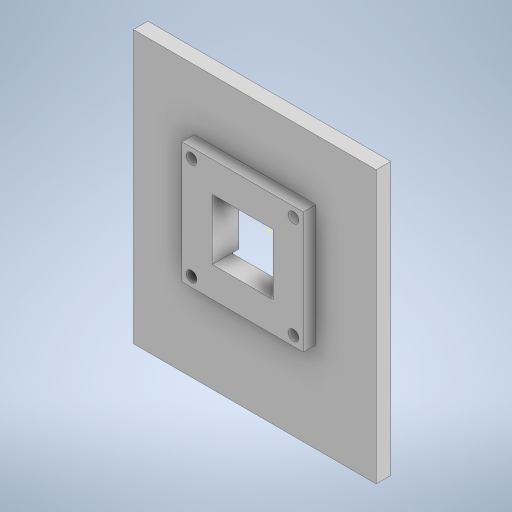
# Autodesk Inventor part: 11
Saved by Autodesk Inventor 2024 (Build 280153000, 153)
## iProperties
Created: 2025-12-09
Part Number: 11
Material: 常规
Document SubType Name: Modeling
Designer: 29555
Density: 1 g/cm^3
Appearance: 默认
Author: 29555
Autodesk Inventor part; units mm, degrees
ref_plane "YZ Plane" through (0, 0, 0) normal (1, 0, 0) x (0, 1, 0)
ref_plane "XZ Plane" through (0, 0, 0) normal (0, 1, 0) x (-1, 0, 0)
ref_plane "XY Plane" through (0, 0, 0) normal (0, 0, 1) x (1, 0, 0)
sketch "草图1" plane through (0, 0, 0) normal (0, 0, 1) x (1, 0, 0)
  line L0 (-50, -50) -> (50, -50)
  line L1 (50, -50) -> (50, 50)
  line L2 (50, 50) -> (-50, 50)
  line L3 (-50, 50) -> (-50, -50)
  line L4 (-50, -50) -> (50, 50) construction
  line L5 (50, -50) -> (-50, 50) construction
  point P0 (0, 0)
  dimension "d0" = 100
  dimension "d1" = 100
  constraints: 12 end point, 2 midpoint, 2 parallel, 1 horizontal, 1 perpendicular
  measures "d0" distance of L1.end L2.end
  measures "d1" distance of L2.end L0.start
extrude "拉伸1" add sketch "草图1" along normal blind 6
sketch "草图2" plane through (0, 0, 6) normal (0, 0, 1) x (1, 0, 0)
  line L0 (-25, -25) -> (25, -25)
  line L1 (25, -25) -> (25, 25)
  line L2 (25, 25) -> (-25, 25)
  line L3 (-25, 25) -> (-25, -25)
  line L4 (-25, -25) -> (25, 25) construction
  line L5 (25, -25) -> (-25, 25) construction
  point P0 (0, 0)
  dimension "d4" = 50
  dimension "d5" = 50
  constraints: 12 end point, 2 midpoint, 2 parallel, 1 horizontal, 1 perpendicular
  measures "d4" distance of L1.end L2.end
  measures "d5" distance of L0.end L1.end
extrude "拉伸2" add sketch "草图2" along normal blind 5
sketch "草图3" plane through (0, 0, 11) normal (0, 0, 1) x (1, 0, 0)
  line L0 (-17.5, -17.5) -> (17.5, -17.5)
  line L1 (17.5, -17.5) -> (17.5, 17.5)
  line L2 (17.5, 17.5) -> (-17.5, 17.5)
  line L3 (-17.5, 17.5) -> (-17.5, -17.5)
  line L4 (-17.5, -17.5) -> (17.5, 17.5) construction
  line L5 (17.5, -17.5) -> (-17.5, 17.5) construction
  point P0 (0, 0)
  dimension "d8" = 35
  dimension "d9" = 35
  constraints: 12 end point, 2 midpoint, 2 parallel, 1 horizontal, 1 perpendicular
  measures "d8" distance of L1.end L2.end
  measures "d9" distance of L0.end L1.end
extrude "拉伸3" cut sketch "草图3" against normal through all
sketch "草图4" plane through (0, 0, 11) normal (0, 0, 1) x (1, 0, 0)
  line L0 (-21, -21) -> (21, -21)
  line L1 (21, -21) -> (21, 21)
  line L2 (21, 21) -> (-21, 21)
  line L3 (-21, 21) -> (-21, -21)
  line L4 (-21, -21) -> (21, 21) construction
  line L5 (21, -21) -> (-21, 21) construction
  circle A0 centre (21, 21) radius 2.15
  circle A1 centre (-21, 21) radius 2.15
  circle A2 centre (21, -21) radius 2.15
  circle A3 centre (-21, -21) radius 2.15
  point P0 (0, 0)
  dimension "d12" = 42
  dimension "d13" = 42
  dimension "d14" = 4.3
  dimension "d15" = 4.3
  dimension "d16" = 4.3
  dimension "d17" = 4.3
  constraints: 12 end point, 4 centre point, 4 coincident, 2 midpoint, 2 parallel, 1 horizontal, 1 perpendicular
  measures "d12" distance of L1.end L2.end
  measures "d13" distance of L0.end L1.end
  measures "d14" diameter of A1
  measures "d15" diameter of A0
  measures "d16" diameter of A3
  measures "d17" diameter of A2
extrude "拉伸4" cut sketch "草图4" against normal through all contours L3 A3 L0 | L0 A3 L3 | A2 L1 L0 | L0 L1 A2 | A1 L2 L3 | L3 L2 A1 | A0 L2 L1 | L1 L2 A0
sketch "草图5" plane through (0, 0, 0) normal (0, 0, -1) x (-1, 0, 0)
  line L0 (15, 22.5) -> (-15, 22.5)
  line L1 (-15, -17.5) -> (-15, -57.5)
  line L2 (-15, -57.5) -> (15, -57.5)
  line L3 (15, -57.5) -> (15, -17.5)
  line L4 (17.5, -17.5) -> (-17.5, -17.5) projected
  line L5 (15, 22.5) -> (-15, -57.5) construction
  line L6 (-15, 22.5) -> (15, -57.5) construction
  line L7 (-15, -17.5) -> (15, -17.5)
  line L8 (12.5, -12.5) -> (-12.5, -12.5)
  line L9 (-12.5, -12.5) -> (-12.5, 12.5)
  line L10 (-12.5, 12.5) -> (12.5, 12.5)
  line L11 (12.5, 12.5) -> (12.5, -12.5)
  line L12 (12.5, -12.5) -> (-12.5, 12.5) construction
  line L13 (-12.5, -12.5) -> (12.5, 12.5) construction
  line L14 (17.5, -17.5) -> (-17.5, -17.5)
  line L15 (-17.5, -17.5) -> (-17.5, 17.5)
  line L16 (-17.5, 17.5) -> (17.5, 17.5)
  line L17 (17.5, 17.5) -> (17.5, -17.5)
  line L18 (17.5, -17.5) -> (-17.5, 17.5) construction
  line L19 (-17.5, -17.5) -> (17.5, 17.5) construction
  point P0 (0, 0)
  point P1 (0, -17.5)
  dimension "d20" = 30
  dimension "d21" = 80
  dimension "d22" = 30
  dimension "d23" = 40
  dimension "d31" = 25
  dimension "d32" = 25
  constraints: 38 end point, 7 midpoint, 6 parallel, 3 horizontal, 3 perpendicular, 3 point on line
  measures "d20" distance of L0.start L0.end
  measures "d21" distance of L2.end L0.start
  measures "d22" distance of L1.end L2.end
  measures "d23" distance of L2.end L3.end
  measures "d31" distance of L9.end L10.end
  measures "d32" distance of L8.end L9.end
sketch "草图6" plane through (-50, -50, 0) normal (0, -1, 0) x (1, 0, 0)
  line L0 (0, 0) -> (0, 6) projected
  line L1 (100, 0) -> (0, 0)
  line L2 (0, 0) -> (0, 6)
  line L3 (0, 6) -> (100, 6)
  line L4 (100, 6) -> (100, 0)
  point P0 (50, 0)
  constraints: 8 end point, 2 parallel, 1 horizontal, 1 perpendicular
extrude "拉伸5" add sketch "草图6" along normal blind 15
sketch "草图7" plane through (0, 0, 0) normal (0, 0, -1) x (-1, 0, 0)
  point P0 (0, 0)
extrude "拉伸6" cut sketch "草图5" against normal blind 3 contours L4 L3 L2 L1
sketch "草图8" plane through (0, 0, 0) normal (0, 0, -1) x (-1, 0, 0)
  line L0 (15, -57.5) -> (-15, -57.5) projected
  line L1 (-9.993, -57.5) -> (10.007, -57.5)
  line L2 (10.007, -57.5) -> (10.007, -69.9689)
  line L3 (10.007, -69.9689) -> (-9.993, -69.9689)
  line L4 (-9.993, -69.9689) -> (-9.993, -57.5)
  line L5 (10.007, -69.9689) -> (0.007, -69.9689)
  point P0 (0, 0)
  dimension "d28" = 20
  constraints: 10 end point, 2 parallel, 1 horizontal, 1 midpoint, 1 perpendicular, 1 point on line
  measures "d28" distance of L2.end L3.end
extrude "拉伸7" cut sketch "草图8" against normal blind 3
sketch "草图9" plane through (0, 0, 11) normal (0, 0, 1) x (1, 0, 0)
  line L0 (17.5, 17.5) -> (17.5, -17.5) projected
  line L1 (-17.5, -17.5) -> (17.5, -17.5)
  line L2 (17.5, -17.5) -> (17.5, 17.5)
  line L3 (17.5, 17.5) -> (-17.5, 17.5)
  line L4 (-17.5, 17.5) -> (-17.5, -17.5)
  line L5 (-17.5, -17.5) -> (17.5, 17.5) construction
  line L6 (17.5, -17.5) -> (-17.5, 17.5) construction
  line L7 (-12.5, -12.5) -> (12.5, -12.5)
  line L8 (12.5, -12.5) -> (12.5, 12.5)
  line L9 (12.5, 12.5) -> (-12.5, 12.5)
  line L10 (-12.5, 12.5) -> (-12.5, -12.5)
  line L11 (-12.5, -12.5) -> (12.5, 12.5) construction
  line L12 (12.5, -12.5) -> (-12.5, 12.5) construction
  point P0 (0, 0)
  dimension "d33" = 25
  dimension "d34" = 25
  constraints: 24 end point, 4 midpoint, 4 parallel, 2 horizontal, 2 perpendicular, 1 point on line
  measures "d33" distance of L8.end L9.end
  measures "d34" distance of L7.end L8.end
extrude "拉伸8" add sketch "草图9" against normal blind 11
sketch "草图10" plane through (0, 0, 0) normal (0, 0, -1) x (-1, 0, 0)
  line L0 (-15, -57.5) -> (-15, -17.5) projected
  line L1 (-15, -17.5) -> (15, -17.5)
  line L2 (15, -17.5) -> (15, -12.5)
  line L3 (15, -12.5) -> (-15, -12.5)
  line L4 (-15, -12.5) -> (-15, -17.5)
  point P0 (0, 0)
  dimension "d37" = 5
  constraints: 8 end point, 2 parallel, 1 horizontal, 1 perpendicular
  measures "d37" distance of L1.end L2.end
extrude "拉伸9" cut sketch "草图10" against normal blind 3
sketch "草图11" plane through (0, 0, 0) normal (0, 0, -1) x (-1, 0, 0)
  line L0 (-50, -65) -> (-50, 50) projected
  line L1 (-50, -65) -> (-34.1728, -65)
  line L2 (-34.1728, -65) -> (-34.1728, -62)
  line L3 (-34.1728, -62) -> (-50, -62)
  line L4 (-50, -62) -> (-50, -65)
  line L5 (50, 50) -> (50, -65) projected
  line L6 (-50, -65) -> (50, -65)
  line L7 (50, -65) -> (50, -62)
  line L8 (50, -62) -> (-50, -62)
  line L9 (-50, -62) -> (-50, -65)
  point P0 (0, 0)
  dimension "d40" = 3
  constraints: 16 end point, 4 parallel, 2 horizontal, 2 perpendicular, 1 point on line
  measures "d40" distance of L1.end L2.end
extrude "拉伸10" cut sketch "草图11" against normal blind 11
